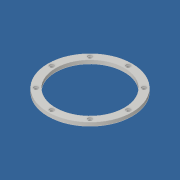
# Autodesk Inventor part: _baseBearingMount
Saved by Autodesk Inventor 2016 (Build 200138000, 138)
## iProperties
Created: 2016-03-04
Part Number: _baseBearingMount
Material: ABS-Kunststoff
Document SubType Name: Modeling
Designer: 4ndreas
Density: 1.06 g/cm^3
Appearance: Glatt - weiß
Mass: 50.4345 g
Surface Area: 214.999 cm^2
Volume: 47.5797 cm^3
Author: 4ndreas
Autodesk Inventor part; units mm, degrees
ref_plane "YZ Plane" through (0, 0, 0) normal (1, 0, 0) x (0, 1, 0)
ref_plane "XZ Plane" through (0, 0, 0) normal (0, 1, 0) x (-1, 0, 0)
ref_plane "XY Plane" through (0, 0, 0) normal (0, 0, 1) x (1, 0, 0)
sketch "Skizze1" plane through (0, 0, 0) normal (0, 0, 1) x (1, 0, 0)
  circle A0 centre (0, 0) radius 67.5
  circle A1 centre (0, 0) radius 82.5
  dimension "d0" = 135
  dimension "d1" = 15
  constraints: 2 centre point, 2 coincident
  measures "d0" diameter of A0
  measures "d1" radial gap between concentric circles of A1 A0
extrude "Extrusion1" add sketch "Skizze1" along normal blind 7
sketch "Skizze2" plane through (0, 0, 7) normal (0, 0, 1) x (1, 0, 0)
  circle A0 centre (0, 0) radius 67.5 projected
  circle A1 centre (0, 0) radius 82.5 projected
  line L0 (0, 0) -> (-82.5, 0) construction
  line L1 (-82.5, 0) -> (-67.5, 0)
  point P0 (-75, 0)
  constraints: 4 end point, 2 horizontal alignment, 1 horizontal, 1 midpoint, 1 point on line, 2 other
hole "Bohrung1" at (-75, 0, 7) direction (0, 0, -1) diameter 5.3 end through all counterbore diameter 9 counterbore depth 2
pattern_circular "Runde Anordnung1" count 8 over 360 about axis through (0, 0, 0) along (0, 0, 1) of "Bohrung1"
